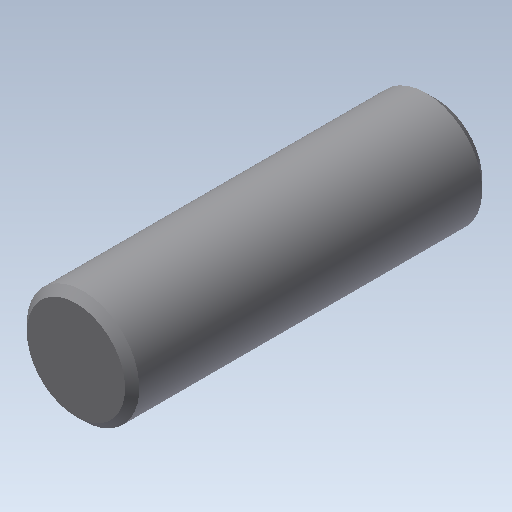
# Autodesk Inventor part: D-787
Saved by Autodesk Inventor 2020 (Build 240168000, 168)
## iProperties
Created: 2020-01-07
Part Number: D-787
Material: Generic
Catalog Web Link: www.cadenas.de
Description: Pin-Original Line - Standard Air Cylinders
Vendor: BIMBA
Document SubType Name: Modeling
Designer: psadmin
Manufacturer: BIMBA
Mass: 0.15599 g
Surface Area: 1.78407 cm^2
Volume: 0.15599 cm^3
Density: 1 g/cm^3
Appearance: PSOLRGB-192-192-192
Category: PARTsolutions
Company: BIMBA
PSOL_IDENT_0: {$CADENAS_DATA\23d-libs\bimba\bimba_brand\bimba_imperial\bimba_full_line\original_line_cylinders\sta
PSOL_IDENT_1: ndard_air_cylinders\pin.prj},147 {VTYP=3D},{NB=D-787},{LINA=D-787},{NN=Pin},{DATE=23.12.2019 10:36:4
PSOL_IDENT_2: 7},{GEOMDATE=15.02.2011 00:00:00},{VERSION=},{LINEID=20},{WBVAR=},{WBNUMERIC=}  {NB=D-787},{LINA=D-7
PSOL_IDENT_3: 87},{KT=DUMMY},{PN=D-787},{DIA=0.15625},{L=0.5000}
NN: Pin
NT: Original Line - Standard Air Cylinders
NB: D-787
NBSYN: $PN.
LINA: D-787
PN: D-787
DIA: 0.15625
L: 0.5
SUPPLIER: BIMBA
ARTICLENO: D-787
BOMINFO: D-787
CREATOR: CADENAS GmbH
Title: D-787
Author: Cadenas PARTsolutions
Comments: Original Line - Standard Air Cylinders
Autodesk Inventor part; units mm, degrees
sketch "Sketch_1" plane through (0, 0, 0) normal (1, 0, 0) x (0, 1, 0)
  line L0 (0, -6.35) -> (0, 6.35)
  line L1 (0, 6.35) -> (1.7329, 6.35)
  line L2 (1.7329, 6.35) -> (1.9844, 6.0986)
  line L3 (1.9844, 6.0986) -> (1.9844, -5.9944)
  line L4 (1.9844, -5.9944) -> (1.6288, -6.35)
  line L5 (1.6288, -6.35) -> (0, -6.35)
  line L6 (0, -6.35) -> (0, 6.35)
  constraints: 14 end point
revolve "Revolution1" add sketch "Sketch_1" angle 360 about axis through (0, 0, -6.35) along (0, 0, -1)
ref_plane "dia1_XY" through (-1.9844, 0, 0) normal (0, 0, 1) x (1, 0, 0)
ref_plane "dia1_YZ" through (-1.9844, 0, 0) normal (1, 0, 0) x (0, 1, 0)
ref_plane "dia1_ZX" through (-1.9844, 0, 0) normal (0, 1, 0) x (0, 0, 1)
ref_plane "dia2_XY" through (1.9844, 0, 0) normal (0, 0, 1) x (1, 0, 0)
ref_plane "dia2_YZ" through (1.9844, 0, 0) normal (1, 0, 0) x (0, 1, 0)
ref_plane "dia2_ZX" through (1.9844, 0, 0) normal (0, 1, 0) x (0, 0, 1)
ref_plane "pin_XY" through (0, 0, 0) normal (0, 0, 1) x (1, 0, 0)
ref_plane "pin_YZ" through (0, 0, 0) normal (1, 0, 0) x (0, 1, 0)
ref_plane "pin_ZX" through (0, 0, 0) normal (0, 1, 0) x (0, 0, 1)
ref_plane "pin1_XY" through (0, 0, 6.35) normal (1, 0, 0) x (0, 0, -1)
ref_plane "pin1_YZ" through (0, 0, 6.35) normal (0, 0, -1) x (0, 1, 0)
ref_plane "pin1_ZX" through (0, 0, 6.35) normal (0, 1, 0) x (1, 0, 0)
ref_plane "pin2_XY" through (0, 0, -6.35) normal (1, 0, 0) x (0, 0, -1)
ref_plane "pin2_YZ" through (0, 0, -6.35) normal (0, 0, -1) x (0, 1, 0)
ref_plane "pin2_ZX" through (0, 0, -6.35) normal (0, 1, 0) x (1, 0, 0)
body "Solid1"
